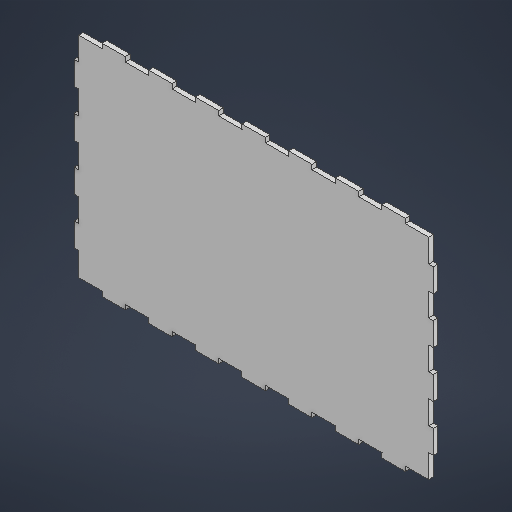
# Autodesk Inventor part: Techo
Saved by Autodesk Inventor 2026 (Build 300175000, 175)
## iProperties
Created: 2026-04-21
Part Number: Techo
Material: Generic
Document SubType Name: Modeling
Designer: juana
Density: 1 g/cm^3
Appearance: Default
Author: juana
Autodesk Inventor part; units mm, degrees
ref_plane "YZ Plane" through (0, 0, 0) normal (1, 0, 0) x (0, 1, 0)
ref_plane "XZ Plane" through (0, 0, 0) normal (0, 1, 0) x (-1, 0, 0)
ref_plane "XY Plane" through (0, 0, 0) normal (0, 0, 1) x (1, 0, 0)
sketch "Sketch1" plane through (0, 0, 0) normal (0, 0, 1) x (1, 0, 0)
  line L0 (0, 135) -> (225, 135)
  line L1 (225, 135) -> (225, 0)
  line L2 (225, 0) -> (0, 0)
  line L3 (0, 0) -> (0, 135)
  dimension "d0" = 135
  dimension "d1" = 225
  constraints: 8 end point, 2 parallel, 1 horizontal, 1 horizontal alignment, 1 perpendicular, 1 vertical alignment
  measures "d0" distance of L0.end L1.end
  measures "d1" distance of L0.start L0.end
extrude "Extrusion1" add sketch "Sketch1" along normal blind 3
sketch "Sketch2" plane through (0, 0, 3) normal (0, 0, 1) x (1, 0, 0)
  line L0 (-3, 120) -> (0, 120)
  line L1 (0, 120) -> (0, 105)
  line L2 (0, 105) -> (-3, 105)
  line L3 (-3, 105) -> (-3, 120)
  line L4 (225, 135) -> (0, 135) projected
  line L5 (-3, 75) -> (-3, 90)
  line L6 (0, 75) -> (-3, 75)
  line L7 (-3, 90) -> (0, 90)
  line L8 (-3, 45) -> (-3, 60)
  line L9 (0, 45) -> (-3, 45)
  line L10 (-3, 60) -> (0, 60)
  line L11 (-3, 15) -> (-3, 30)
  line L12 (0, 15) -> (-3, 15)
  line L13 (-3, 30) -> (0, 30)
  line L14 (225, 105) -> (225, 120)
  line L15 (228, 105) -> (225, 105)
  line L16 (225, 120) -> (228, 120)
  line L17 (225, 75) -> (225, 90)
  line L18 (228, 75) -> (225, 75)
  line L19 (225, 90) -> (228, 90)
  line L20 (225, 45) -> (225, 60)
  line L21 (228, 45) -> (225, 45)
  line L22 (225, 60) -> (228, 60)
  line L23 (225, 15) -> (225, 30)
  line L24 (228, 15) -> (225, 15)
  line L25 (225, 30) -> (228, 30)
  line L26 (228, 120) -> (228, 105)
  line L27 (228, 90) -> (228, 75)
  line L28 (228, 60) -> (228, 45)
  line L29 (228, 30) -> (228, 15)
  line L30 (0, 75) -> (0, 90)
  line L31 (0, 135) -> (0, 0) projected
  line L32 (0, 15) -> (0, 30)
  line L33 (0, 45) -> (0, 60)
  dimension "d4" = 3
  dimension "d5" = 15
  dimension "d6" = 15
  dimension "d9" = 30
  dimension "d12" = 228
  constraints: 64 end point, 5 vertical, 3 collinear, 2 horizontal, 2 parallel, 1 perpendicular, 1 vertical alignment, 50 other
  measures "d4" distance of L0.start L0.end
  measures "d5" distance of L2.end L0.start
  measures "d6" distance from line of L4 L0.end
  measures "d9" distance of L2.end L5.start
  measures "d12" distance of L2.end L14.start
extrude "Extrusion2" add sketch "Sketch2" against normal blind 3
sketch "Sketch3" plane through (0, 0, 3) normal (0, 0, 1) x (1, 0, 0)
  line L0 (225, 135) -> (0, 135) construction
  line L1 (15, 138) -> (30, 138)
  line L2 (30, 138) -> (30, 135)
  line L3 (30, 135) -> (15, 135)
  line L4 (15, 135) -> (15, 138)
  line L5 (60, 135) -> (45, 135)
  line L6 (45, 138) -> (60, 138)
  line L7 (60, 138) -> (60, 135)
  line L8 (45, 135) -> (45, 138)
  line L9 (90, 135) -> (75, 135)
  line L10 (75, 138) -> (90, 138)
  line L11 (90, 138) -> (90, 135)
  line L12 (75, 135) -> (75, 138)
  line L13 (120, 135) -> (105, 135)
  line L14 (105, 138) -> (120, 138)
  line L15 (120, 138) -> (120, 135)
  line L16 (105, 135) -> (105, 138)
  line L17 (150, 135) -> (135, 135)
  line L18 (135, 138) -> (150, 138)
  line L19 (150, 138) -> (150, 135)
  line L20 (135, 135) -> (135, 138)
  line L21 (180, 135) -> (165, 135)
  line L22 (165, 138) -> (180, 138)
  line L23 (180, 138) -> (180, 135)
  line L24 (165, 135) -> (165, 138)
  line L25 (210, 135) -> (195, 135)
  line L26 (195, 138) -> (210, 138)
  line L27 (210, 138) -> (210, 135)
  line L28 (195, 135) -> (195, 138)
  line L29 (0, 135) -> (0, 120) construction
  line L30 (30, -3) -> (15, -3)
  line L31 (15, 0) -> (30, 0)
  line L32 (30, 0) -> (30, -3)
  line L33 (15, -3) -> (15, 0)
  line L34 (60, -3) -> (45, -3)
  line L35 (45, 0) -> (60, 0)
  line L36 (60, 0) -> (60, -3)
  line L37 (45, -3) -> (45, 0)
  line L38 (90, -3) -> (75, -3)
  line L39 (75, 0) -> (90, 0)
  line L40 (90, 0) -> (90, -3)
  line L41 (75, -3) -> (75, 0)
  line L42 (120, -3) -> (105, -3)
  line L43 (105, 0) -> (120, 0)
  line L44 (120, 0) -> (120, -3)
  line L45 (105, -3) -> (105, 0)
  line L46 (150, -3) -> (135, -3)
  line L47 (135, 0) -> (150, 0)
  line L48 (150, 0) -> (150, -3)
  line L49 (135, -3) -> (135, 0)
  line L50 (180, -3) -> (165, -3)
  line L51 (165, 0) -> (180, 0)
  line L52 (180, 0) -> (180, -3)
  line L53 (165, -3) -> (165, 0)
  line L54 (210, -3) -> (195, -3)
  line L55 (195, 0) -> (210, 0)
  line L56 (210, 0) -> (210, -3)
  line L57 (195, -3) -> (195, 0)
  point P0 (0, 0)
  dimension "d17" = 15
  dimension "d18" = 3
  dimension "d19" = 15
  dimension "d22" = 30
  dimension "d25" = 138
  constraints: 112 end point, 2 horizontal, 2 parallel, 1 perpendicular, 1 point on line, 1 vertical, 104 other
  measures "d17" distance of L1.start L1.end
  measures "d18" distance of L1.end L2.end
  measures "d19" distance from line of L0.end L4
  measures "d22" distance of L2.end L5.start
  measures "d25" distance of L2.end L30.start
extrude "Extrusion3" add sketch "Sketch3" against normal blind 3
body "Solid1"
